Autodesk Fusion 360 part; units mm, degrees
(part 3 of 3)
  spline S186 degree 3 poles (-8.1133, -5.6669) (-8.4073, -5.4939) (-8.7359, -5.1307) (-8.8743, -4.8713) knots 0 0 0 0 1 1 1 1
  line L21 (-8.8743, -4.8713) -> (-9.1164, -4.4043)
  line L22 (-9.1164, -4.4043) -> (-8.5457, -4.5254)
  spline S187 degree 3 poles (-8.5457, -4.5254) (-8.2171, -4.5772) (-7.923, -4.7329) (-7.8885, -4.854) knots 0 0 0 0 1 1 1 1
  spline S188 degree 3 poles (-7.8885, -4.854) (-7.8539, -4.9577) (-7.5944, -5.2691) (-7.335, -5.5285) knots 0 0 0 0 1 1 1 1
  spline S189 degree 3 poles (-7.335, -5.5285) (-6.8853, -5.9955) (-6.868, -6.0128) (-7.2312, -6.0128) knots 0 0 0 0 1 1 1 1
  spline S190 degree 3 poles (-7.2312, -6.0128) (-7.4388, -6.0128) (-7.8366, -5.8571) (-8.1133, -5.6669) knots 0 0 0 0 1 1 1 1
sketch "Sketch5" plane through (0, -2, 0) normal (0, -1, 0) x (1, 0, 0)
  line L0 (-2.8686, -21.662) -> (5.9996, -21.662)
  line L1 (5.9996, -21.662) -> (5.9996, -34.2128)
  line L2 (5.9996, -34.2128) -> (-2.8686, -34.2128)
  line L3 (-2.8686, -34.2128) -> (-2.8686, -21.662)
  line L4 (12.3869, -18.9733) -> (18.9543, -18.9733)
  line L5 (18.9543, -18.9733) -> (18.9543, -21.1268)
  line L6 (18.9543, -21.1268) -> (12.3869, -21.1268)
  line L7 (12.3869, -21.1268) -> (12.3869, -18.9733)
  line L8 (-9.7333, -18.976) -> (-16.4295, -18.976)
  line L9 (-16.4295, -18.976) -> (-16.4295, -21.1436)
  line L10 (-16.4295, -21.1436) -> (-9.7333, -21.1436)
  line L11 (-9.7333, -21.1436) -> (-9.7333, -18.976)
  line L12 (10.1555, -10.4776) -> (19, -10.4776)
  line L13 (19, -10.4776) -> (19, -12.5659)
  line L14 (19, -12.5659) -> (10.1555, -12.5659)
  line L15 (10.1555, -12.5659) -> (10.1555, -10.4776)
  line L16 (-7.0448, -10.4497) -> (-17.0149, -10.4497)
  line L17 (-17.0149, -10.4497) -> (-17.0149, -12.6031)
  line L18 (-17.0149, -12.6031) -> (-7.0448, -12.6031)
  line L19 (-7.0448, -12.6031) -> (-7.0448, -10.4497)
  spline S0 degree 3 poles (-2.4577, -9.8869) (-4.9309, -10.0599) (-7.6463, -10.475) (-8.1825, -10.7517) knots 0 0 0 0 1 1 1 1
  line L20 (-7.7381, 5.4735) -> (-14.5, 15)
  line L21 (-14.5, 15) -> (-10.5, 17.5)
  line L22 (-10.5, 17.5) -> (-5.5, 17.5)
  line L23 (-5.5, 17.5) -> (0.2898, 8.079)
  line L24 (0.2898, 8.079) -> (-7.7381, 5.4735)
  line L25 (6.5, 5.4735) -> (15.2622, 17.5)
  line L26 (15.2622, 17.5) -> (19.9656, 11.4868)
  line L27 (19.9656, 11.4868) -> (19, 6.5)
  line L28 (19, 6.5) -> (12.3493, 3.6465)
  line L29 (12.3493, 3.6465) -> (9.8938, 5.0732)
  line L30 (9.8938, 5.0732) -> (6.5, 5.4735)
  line L31 (13.2195, 0.2063) -> (19, 0.2063)
  line L32 (19, 0.2063) -> (19, -3.3977)
  line L33 (19, -3.3977) -> (13.2195, -3.3977)
  line L34 (13.2195, -3.3977) -> (13.2195, 0.2063)
  line L35 (-10.5, 1.1733) -> (-17, 1.1733)
  line L36 (-17, 1.1733) -> (-17, -2.8416)
  line L37 (-17, -2.8416) -> (-10.5, -2.8416)
  line L38 (-10.5, -2.8416) -> (-10.5, 1.1733)
  constraint horizontal L0
  constraint vertical L1
  constraint horizontal L2
  constraint vertical L3
  constraint horizontal L4
  constraint vertical L5
  constraint horizontal L6
  constraint vertical L7
  constraint horizontal L8
  constraint vertical L9
  constraint horizontal L10
  constraint vertical L11
  constraint horizontal L12
  constraint vertical L13
  constraint horizontal L14
  constraint vertical L15
  constraint horizontal L16
  constraint vertical L17
  constraint horizontal L18
  constraint vertical L19
  constraint coincident L16.start S0
  constraint horizontal L22
  constraint horizontal L31
  constraint vertical L32
  constraint horizontal L33
  constraint vertical L34
  constraint horizontal L35
  constraint vertical L36
  constraint horizontal L37
  constraint vertical L38
extrude "Extrude5" add sketch "Sketch5" sketch "Sketch4" 1 faces at (-17.7069, -2, -16.2923) along normal blind 5 of sketch 2 on bodies 2 bodies 1 2
